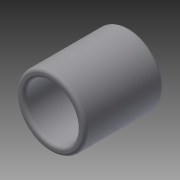
# Autodesk Inventor part: Spacer
Saved by Autodesk Inventor 2014 (Build 180170000, 170)
## iProperties
Created: 2015-02-08
Part Number: Spacer
Material: Generic
Document SubType Name: Modeling
Designer: Spooner
Density: 1 g/cm^3
Appearance: Default
Author: Spooner
Autodesk Inventor part; units mm, degrees
ref_plane "YZ Plane" through (0, 0, 0) normal (1, 0, 0) x (0, 1, 0)
ref_plane "XZ Plane" through (0, 0, 0) normal (0, 1, 0) x (-1, 0, 0)
ref_plane "XY Plane" through (0, 0, 0) normal (0, 0, 1) x (1, 0, 0)
sketch "Sketch1" plane through (0, 0, 0) normal (0, 0, 1) x (1, 0, 0)
  circle A0 centre (0, 0) radius 6.6675
  circle A1 centre (0, 0) radius 5.08
  dimension "d0" = 13.335
  dimension "d1" = 10.16
  constraints: 2 centre point, 2 coincident
  measures "d0" diameter of A0
  measures "d1" diameter of A1
extrude "Extrusion1" add sketch "Sketch1" along normal blind 15.24
fillet "Fillet1" radius 0.635 4 edges at (-6.6675, 0, 15.24) (-5.08, 0, 15.24) (-6.6675, 0, 0) (-5.08, 0, 0)
body "Solid1"
